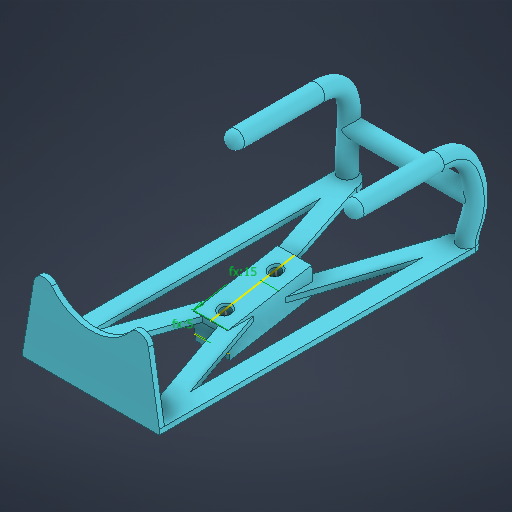
# Autodesk Inventor part: my_portafilter_holder_8
Saved by Autodesk Inventor 2026 (Build 300175000, 175)
## iProperties
Created: 2025-05-06
Part Number: my_portafilter_holder_8
Material: Generic
Document SubType Name: Modeling
Designer: Paul Juschitz
Density: 1 g/cm^3
Appearance: Cadet Blue
Author: Paul Juschitz
Autodesk Inventor part; units mm, degrees
ref_plane "XZ Plane" through (0, 0, 0) normal (0, 1, 0) x (-1, 0, 0)
sketch "Sketch1" plane through (0, 0, 0) normal (0, 1, 0) x (-1, 0, 0)
  line L0 (20, 47.5) -> (-20, 47.5)
  line L1 (-20, 47.5) -> (-20, -47.5)
  line L2 (-20, -47.5) -> (20, -47.5)
  line L3 (20, -47.5) -> (20, 47.5)
  line L4 (20, 47.5) -> (-20, -47.5) construction
  line L5 (-20, 47.5) -> (20, -47.5) construction
  point P0 (0, 0)
  dimension "holder_width" = 40
  dimension "holder_length" = 95
  constraints: 12 end point, 2 midpoint, 2 parallel, 1 horizontal, 1 perpendicular
  measures "holder_width" distance of L2.end L1.end
  measures "holder_length" distance of L1.end L0.end
extrude "Extrusion1" add sketch "Sketch1" along normal blind 1.5
sketch "Sketch2" plane through (0, 1.5, 0) normal (0, 1, 0) x (1, 0, 0)
  line L0 (-20, 47.5) -> (-20, -47.5) projected
  line L1 (20, -47.5) -> (20, 47.5) projected
  line L2 (-20, -47.5) -> (20, -47.5)
  line L3 (20, -47.5) -> (20, -46)
  line L4 (20, -46) -> (-20, -46)
  line L5 (-20, -46) -> (-20, -47.5)
  point P0 (0, 0)
  point P1 (-20, -46)
  dimension "d4" = 1.5
  constraints: 8 end point, 2 parallel, 1 horizontal, 1 perpendicular, 1 point on line
  measures "d4" distance of L3.end L2.end
extrude "Extrusion2" add sketch "Sketch2" along normal blind 25
sketch "Sketch3" plane through (0, 1.5, 0) normal (0, 1, 0) x (1, 0, 0)
  circle A0 centre (17.5, 45) radius 2.5
  line L0 (20, 47.5) -> (-20, 47.5) projected
  line L1 (20, -46) -> (20, 47.5) projected
  point P0 (0, 0)
  dimension "prong_diameter" = 5
  constraints: 2 tangent, 1 centre point
  measures "prong_diameter" diameter of A0
sketch3d "3D Sketch1"
  spline S0 degree 4 poles (17.5, 1.5, -45) (17.5, 5.5, -45) (20, 9.5, -47.5) (17.5, 21.5, -47.5) (17.5, 26.5, -42) (17.5, 26.5, -36) knots 1 1 1 1 1 2 3 3 3 3 3
  line L0 (17.5, 26.5, -36) -> (17.5, 26.5, -10.0001)
  dimension "d14" = 35
  dimension "d15" = 8
  dimension "d16" = 20
  dimension "d17" = 6
  dimension "d18" = 9
  dimension "d19" = 4
  dimension "prong_height" = 25
  dimension "prong_length" = 34.9999
sweep "Sweep1" add profiles "Sketch3" path "3D Sketch1" contours A0
fillet "Fillet1" radius 2.5 1 edges at (15.0105, 26.2713, -10.0001)
mirror "Mirror1" about plane through (0, 0, 0) normal (1, 0, 0) of "Fillet1", "Sweep1"
sketch "Sketch5" plane through (0, 1.5, 0) normal (0, 1, 0) x (1, 0, 0)
  line L0 (17.5, 47.5) -> (-17.5, 47.5) construction
  line L1 (-20, 45) -> (-20, -46) construction
  line L2 (20, -46) -> (-20, -46) construction
  line L3 (20, -46) -> (20, 45) construction
  line L4 (20, 45) -> (20, 47.5) construction
  line L5 (20, 47.5) -> (17.5, 47.5) construction
  line L6 (-17.5, 47.5) -> (-20, 47.5) construction
  line L7 (-20, 47.5) -> (-20, 45) construction
  line L8 (-20, 47.5) -> (20, 47.5)
  line L9 (20, 47.5) -> (20, -46)
  line L10 (20, -46) -> (-20, -46)
  line L11 (-20, -46) -> (-20, 47.5)
  line L12 (-15, -41) -> (-15, 42.5) construction
  line L13 (-15, 42.5) -> (15, 42.5) construction
  line L14 (15, 42.5) -> (15, -41) construction
  line L15 (15, -41) -> (-15, -41) construction
  line L16 (0, 47.5) -> (0, -46)
  line L17 (-5, 12.5) -> (5, 12.5) construction
  line L18 (5, 12.5) -> (5, -12.5) construction
  line L19 (5, -12.5) -> (-5, -12.5) construction
  line L20 (-5, -12.5) -> (-5, 12.5) construction
  line L21 (-5, 12.5) -> (5, -12.5) construction
  line L22 (5, 12.5) -> (-5, -12.5) construction
  line L23 (15, 34.5943) -> (5, 4.5943)
  line L24 (12.3648, 42.5) -> (2.3648, 12.5)
  line L25 (15, 42.5) -> (5, 12.5) construction
  line L26 (15, -33.4491) -> (5, -4.9491)
  line L27 (12.3506, -41) -> (2.3506, -12.5)
  line L28 (15, -41) -> (5, -12.5) construction
  line L29 (-15, 34.5943) -> (-5, 4.5943)
  line L30 (-12.3648, 42.5) -> (-2.3648, 12.5)
  line L31 (-15, 42.5) -> (-5, 12.5) construction
  line L32 (-15, -33.4491) -> (-5, -4.9491)
  line L33 (-12.3506, -41) -> (-2.3506, -12.5)
  line L34 (-15, -41) -> (-5, -12.5) construction
  line L35 (-2.3648, 12.5) -> (2.3648, 12.5)
  line L36 (5, 4.5943) -> (5, -4.9491)
  line L37 (2.3506, -12.5) -> (-2.3506, -12.5)
  line L38 (-5, 4.5943) -> (-5, -4.9491)
  line L39 (-15, 34.5943) -> (-15, -33.4491)
  line L40 (-12.3506, -41) -> (12.3506, -41)
  line L41 (15, -33.4491) -> (15, 34.5943)
  line L42 (12.3648, 42.5) -> (-12.3648, 42.5)
  point P0 (0, 0)
  point P1 (0, 0)
  dimension "d34" = 5
  dimension "d35" = 10
  dimension "d36" = 25
  dimension "d37" = 35
  dimension "d38" = 5
  dimension "d39" = 5
  constraints: 70 end point, 9 point on line, 8 symmetric about line, 6 parallel, 4 collinear, 4 midpoint, 4 perpendicular, 3 horizontal, 1 vertical, 5 other
  measures "d34" distance between parallel lines of L1 L12
  measures "d35" distance of L18.end L19.end
  measures "d36" distance between parallel lines of L17 L19
  measures "d37" distance between parallel lines of L0 L17
  measures "d38" distance between parallel lines of L23 L24
  measures "d39" distance between parallel lines of L26 L27
extrude "Extrusion3" cut sketch "Sketch5" against normal up to surface (1.5 mm away) contours L42 L24 L35 L16 | L16 L35 L30 L42 | L40 L33 L37 L16 | L16 L37 L27 L40 | L41 L26 L36 L23 | L29 L38 L32 L39
sketch "Sketch8" plane through (-20, 0, 47.5) normal (0, 0, 1) x (1, 0, 0)
  arc A0 (8.5, 22.0557) -> (3.1867, 20.6595) centre (6.1499, 20.1911) ccw
  arc A1 (8.5, 22.0557) -> (31.5, 22.0557) centre (20, 31.18) ccw
  arc A2 (36.8095, 20.6833) -> (31.5, 22.0557) centre (33.8501, 20.1911) ccw
  line L0 (20, 0) -> (20, 47.7301)
  circle A3 centre (37.5, 26.5) radius 2.5 construction
  line L1 (20, 16.5) -> (37.5, 16.5) construction
  line L2 (37.5, 16.5) -> (37.5, 29) construction
  line L3 (0, 1.5) -> (40, 1.5) construction
  line L4 (40, 0) -> (40, 1.5) projected
  line L5 (40, 0) -> (40, 1.5)
  line L6 (40, 1.5) -> (36.8095, 20.6833)
  line L7 (0, 0) -> (0, 1.5)
  line L8 (0, 1.5) -> (3.1905, 20.6833)
  line L9 (0, 0) -> (0, 26.5) projected
  line L10 (0, 26.5) -> (40, 26.5) projected
  line L11 (40, 0) -> (40, 26.5) projected
  point P0 (3.1905, 20.6833)
  dimension "basket_handle_height" = 12.5
  dimension "d54" = 14.68
  dimension "d55" = 3
  dimension "d56" = 23
  constraints: 14 end point, 8 point on circle, 3 centre point, 3 tangent, 2 symmetric about line, 1 collinear, 1 equal radius, 1 horizontal, 1 line through centre, 1 perpendicular, 1 point on line, 1 vertical, 1 other
  measures "basket_handle_height" distance of L1.end L2.end
  measures "d54" radius of A1
  measures "d55" radius of A2
  measures "d56" distance of A1.end A0.start
extrude "Extrusion5" cut sketch "Sketch8" against normal up to surface (1.5 mm away)
sketch "Sketch9" plane through (0, 0, 0) normal (0, -1, 0) x (1, 0, 0)
  line L0 (5, 12.5) -> (-5, 12.5)
  line L1 (-5, 12.5) -> (-5, -12.5)
  line L2 (-5, -12.5) -> (5, -12.5)
  line L3 (5, -12.5) -> (5, 12.5)
  point P0 (0, 0)
  point P1 (2.3506, 12.5)
  point P2 (-2.3506, 12.5)
  point P3 (-5, 4.9491)
  point P4 (-5, -4.5943)
  point P5 (-2.3648, -12.5)
  point P6 (2.3648, -12.5)
  point P7 (5, -4.5943)
  point P8 (5, 4.9491)
  constraints: 8 end point, 4 point on line, 2 parallel, 1 horizontal, 1 perpendicular
extrude "Extrusion6" add sketch "Sketch9" along normal blind 0.1
sketch "Sketch10" plane through (0, -0.1, 0) normal (0, -1, 0) x (1, 0, 0)
  line L0 (-5, 12.5) -> (-5, -12.5) projected
  line L1 (-5, -12.5) -> (5, -12.5) projected
  line L2 (5, -12.5) -> (5, 12.5) projected
  line L3 (5, 12.5) -> (-5, 12.5) projected
  point P0 (0, 0)
revolve "Revolution1" add sketch "Sketch10" angle 10 about axis through (-5, -0.1, -12.5) along (1, 0, 0)
sketch "Sketch11" plane through (-5, -0.1, -12.5) normal (0, -0.9848078, -0.1736482) x (1, 0, 0)
  line L0 (0, 0) -> (10, 0) construction
  line L1 (5, 0) -> (5, 25)
  line L2 (10, 25) -> (0, 25) projected
  point P0 (5, 12.2927)
  point P1 (5, 5)
  point P2 (5, 20)
  point P3 (5, 25)
  dimension "d62" = 5
  dimension "d63" = 15
  constraints: 3 midpoint, 2 end point, 2 point on line, 1 vertical
  measures "d62" distance of point (5, 25) point (5, 20)
  measures "d63" distance of point (5, 5) point (5, 20)
sketch "Sketch13" plane through (0, 1.5, 0) normal (0, 1, 0) x (1, 0, 0)
  line L0 (5, -12.5) -> (5, -4.9491) projected
  line L1 (-2.3648, 12.5) -> (-5, 12.5) projected
  line L2 (5, -12.5) -> (-5, -12.5)
  line L3 (-5, -12.5) -> (-5, 12.5)
  line L4 (-5, 12.5) -> (5, 12.5)
  line L5 (5, 12.5) -> (5, -12.5)
  point P0 (0, 0)
  point P1 (2.3506, -12.5)
  point P2 (2.3648, 12.5)
  point P3 (-5, 4.5943)
  point P4 (5, -4.9491)
  constraints: 8 end point, 2 parallel, 1 horizontal, 1 perpendicular
revolve "Revolution2" add sketch "Sketch13" angle 10 about axis through (5, 1.5, 12.5) along (1, 0, 0)
sketch "Sketch14" plane through (0, 0, 0) normal (1, 0, 0) x (0, 1, 0)
  line L0 (-0.9682, -7.576) -> (4.8588, -6.5485)
  line L1 (1.5, 12.5) -> (5.8412, -12.1202) projected
  line L2 (-3.573, 7.1962) -> (1.5105, 8.0925)
  line L3 (-0.1, -12.5) -> (-4.4412, 12.1202) projected
  point P0 (0, 0)
  constraints: 4 end point, 1 parallel, 1 perpendicular, 1 point on line
sketch "Sketch15" plane through (-5, 1.5, 12.5) normal (0, 0.9848078, 0.1736482) x (1, 0, 0)
  point P0 (5, 12.0496)
  point P1 (5, 4.3424)
  point P2 (5, 19.3424)
sketch "Sketch16" plane through (-5, -0.1, -12.5) normal (0, -0.9848078, -0.1736482) x (1, 0, 0)
  line L0 (0, 0) -> (10, 0) projected
  line L1 (10, 0) -> (10, 25) projected
  line L2 (10, 25) -> (0, 25) projected
  line L3 (0, 25) -> (0, 0) projected
  point P0 (5, 12.2927)
extrude "Extrusion7" add sketch "Sketch16" along normal blind 2
hole "Hole3" at (0, 2.254, 8.2236) at (0, 4.8588, -6.5485) direction (0, -0.9848078, -0.1736482) diameter 3 end through all countersink diameter 4 countersink angle 90
ref_plane "Work Plane1" through (-20, 0.75, 47.5) normal (1, 0, 0) x (0, 1, 0)
sketch "Sketch17" plane through (0, 0, 0) normal (1, 0, 0) x (0, 1, 0)
  line L0 (1.5, -47.5) -> (1.5, -45) construction
  line L1 (1.5, -45) -> (1.5, -47.5) construction
  line L2 (29, -36) -> (24, -36) construction
  circle A0 centre (12.5, -46.6061) radius 2.5
  point P0 (0, 0)
  dimension "d81" = 5
  dimension "d82" = 11
  constraints: 1 centre point, 2 other
  measures "d81" diameter of A0
  measures "d82" horizontal distance of L0.end A0.centre
ref_plane "Work Plane2" through (0, 12.5, -46.6061) normal (0, 0, 1) x (1, 0, 0)
sketch "Sketch18" plane through (0, 12.5, -46.6061) normal (0, 0, 1) x (1, 0, 0)
  line L0 (17.5, -11) -> (20, -11) construction
  line L1 (20, -11) -> (17.5, -11) construction
  circle A0 centre (17.5, 14) radius 2.5 construction
  line L2 (0, 0) -> (21.0869, 0) construction
  line L3 (0, 0) -> (18.5869, 0)
  point P0 (0, -12.5)
  dimension "d85" = 2.5
  constraints: 4 end point, 1 horizontal, 1 point on line, 3 other
  measures "d85" distance of L2.end L3.end
sweep "Sweep2" add profiles "Sketch17" path "Sketch18"
mirror "Mirror2" about plane through (0, 0, 0) normal (1, 0, 0) of "Sweep2"
sketch "Sketch19" plane through (0, 0, 0) normal (0, -1, 0) x (1, 0, 0)
  line L0 (-12.3648, -42.5) -> (12.3648, -42.5) construction
  line L1 (17.5, -47.5) -> (-17.5, -47.5) construction
  line L2 (20, -47.5) -> (-20, -47.5) construction
  line L3 (12.3648, -42.5) -> (-12.3648, -42.5)
  line L4 (-12.3648, -42.5) -> (-12.3648, -47.5) construction
  line L5 (-12.3648, -47.5) -> (12.3648, -47.5) construction
  line L6 (12.3648, -47.5) -> (12.3648, -42.5) construction
  arc A0 (12.3648, -42.5) -> (17.5, -47.5) centre (17.3665, -42.5) ccw
  line L7 (17.5, -47.5) -> (-17.5, -47.5)
  arc A1 (-17.5, -47.5) -> (-12.3648, -42.5) centre (-17.5, -42.3629) ccw
  point P0 (0, 0)
  point P1 (17.2331, -47.5)
  constraints: 10 end point, 4 point on circle, 2 centre point, 2 parallel, 1 collinear, 1 horizontal, 1 perpendicular, 1 point on line, 1 tangent, 4 other
extrude "Extrusion8" cut sketch "Sketch19" against normal up to surface (1.5 mm away)
fillet "Fillet2" radius 2.5 2 edges at (20, 0.75, -47.5) (-20, 0.75, -47.5)
ref_plane "Work Plane3" through (0, 0, 0) normal (1, 0, 0) x (0, 1, 0)
equation "\"d4\" = print_thickness_1"
equation "\"d22\" = 0.5 * prong_diameter"
equation "\"d34\" = prong_diameter"
equation "\"d35\" = load_cell_width"
equation "\"d37\" = holder_load_cell_setback"
equation "\"d38\" = prong_diameter"
equation "\"d39\" = prong_diameter"
equation "\"d54\" = handle_radius"
equation "\"d62\" = load_cell_hole_inset"
equation "\"d63\" = load_cell_hole_spacing"
equation "\"d64\" = holder_angle"
equation "\"d81\" = prong_diameter"
equation "\"d85\" = 0.5 * prong_diameter"
equation "\"d88\" = 0.5 * prong_diameter"
equation "\"handle_circumference\" = 92.237"
equation "\"handle_radius\" = 0.159155 * handle_circumference"
equation "\"print_thickness_1\" = 1.5"
equation "\"load_cell_width\" = 10"
equation "\"holder_load_cell_setback\" = 35"
equation "\"holder_angle\" = 10deg"
equation "\"load_cell_hole_inset\" = 5"
equation "\"load_cell_hole_spacing\" = 15"
body "Solid1"
